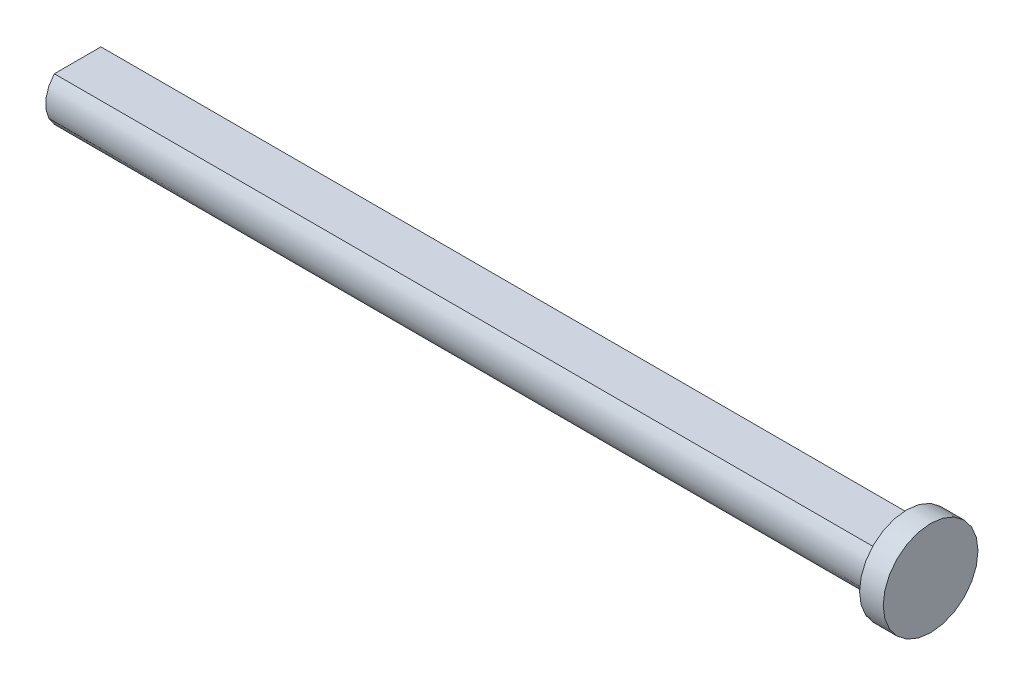
# Autodesk Inventor part: Axle
Saved by Autodesk Inventor 2023.4 (Build 274418000, 418)
## iProperties
Created: 2026-03-03
Part Number: Axle
Material: Generic
Document SubType Name: Modeling
Designer: 1017208
Density: 1 g/cm^3
Appearance: Default
Author: 1017208
## iProperties of the stored document Axle_3DPrint.ipt
Created: 2026-03-03
Part Number: Axle_3DPrint
Material: Generic
Document SubType Name: Modeling
Designer: 1017208
Density: 1 g/cm^3
Appearance: Default
Author: 1017208
Autodesk Inventor part; units mm, degrees
ref_plane "YZ Plane" through (0, 0, 0) normal (1, 0, 0) x (0, 1, 0)
ref_plane "XZ Plane" through (0, 0, 0) normal (0, 1, 0) x (-1, 0, 0)
ref_plane "XY Plane" through (0, 0, 0) normal (0, 0, 1) x (1, 0, 0)
sketch "Sketch1" plane through (0, 0, 0) normal (1, 0, 0) x (0, 1, 0)
  circle A0 centre (0, 0) radius 2.7
  line L0 (-1.85, -2.7) -> (1.85, -2.7)
  line L1 (1.85, -2.7) -> (1.85, 2.7)
  line L2 (1.85, 2.7) -> (-1.85, 2.7)
  line L3 (-1.85, 2.7) -> (-1.85, -2.7)
  line L4 (-1.85, -2.7) -> (1.85, 2.7) construction
  line L5 (1.85, -2.7) -> (-1.85, 2.7) construction
  point P0 (-1.85, 1.9666)
  point P1 (-1.85, -1.9666)
  point P2 (1.85, -1.9666)
  point P3 (1.85, 1.9666)
  dimension "d0" = 5.4
  dimension "d1" = 3.7
  dimension "d2" = 5.4
  constraints: 12 end point, 2 midpoint, 2 parallel, 1 centre point, 1 coincident, 1 horizontal, 1 perpendicular
  measures "d0" diameter of A0
  measures "d1" distance of L2.end L1.end
  measures "d2" distance of L1.end L0.end
extrude "Extrusion1" add sketch "Sketch1" against normal blind 70 contours L1 A0 L3
sketch "Sketch2" plane through (0, 0, 0) normal (1, 0, 0) x (0, 0, -1)
  circle A0 centre (0, 0) radius 4
  constraints: 1 centre point, 1 coincident
extrude "Extrusion2" add sketch "Sketch2" along normal blind 2
body "Solid1"
